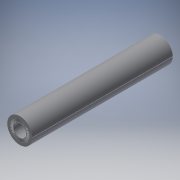
# Autodesk Inventor part: shtamp
Saved by Autodesk Inventor 2016 SP1 (Build 200210100, 210)
## iProperties
Created: 2017-07-05
Part Number: shtamp
Material: Типовые
Document SubType Name: Modeling
Designer: user
Density: 1 g/cm^3
Appearance: По умолчанию
Author: user
Autodesk Inventor part; units mm, degrees
ref_plane "YZ Plane" through (0, 0, 0) normal (1, 0, 0) x (0, 1, 0)
ref_plane "XZ Plane" through (0, 0, 0) normal (0, 1, 0) x (-1, 0, 0)
ref_plane "XY Plane" through (0, 0, 0) normal (0, 0, 1) x (1, 0, 0)
sketch "Эскиз1" plane through (0, 0, 0) normal (0, 1, 0) x (-1, 0, 0)
  arc A0 (-177.7324, -2.5) -> (-177.7324, 2.5) centre (0, 0) ccw
  circle A1 centre (0, 0) radius 90.075
  line L0 (134.775, -4.8) -> (97.375, -4.8)
  line L1 (92.575, 0) -> (92.575, 0)
  line L2 (97.375, 4.8) -> (134.775, 4.8)
  line L3 (139.575, 0) -> (139.575, 0)
  arc A2 (139.575, 0) -> (134.775, 4.8) centre (134.775, 0) ccw
  arc A3 (134.775, -4.8) -> (139.575, 0) centre (134.775, 0) ccw
  arc A4 (97.375, 4.8) -> (92.575, 0) centre (97.375, 0) ccw
  arc A5 (92.575, 0) -> (97.375, -4.8) centre (97.375, 0) ccw
  line L4 (95.9154, 17.4689) -> (132.9955, 22.3506)
  arc A6 (95.9154, 17.4689) -> (91.783, 12.0835) centre (96.5419, 12.71) ccw
  arc A7 (91.783, 12.0835) -> (97.1685, 7.9511) centre (96.5419, 12.71) ccw
  line L5 (134.2485, 12.8327) -> (97.1685, 7.9511)
  arc A8 (134.2485, 12.8327) -> (138.3809, 18.2182) centre (133.622, 17.5917) ccw
  arc A9 (138.3809, 18.2182) -> (132.9955, 22.3506) centre (133.622, 17.5917) ccw
  line L6 (92.8147, 29.8389) -> (128.9403, 39.5188)
  arc A10 (92.8147, 29.8389) -> (89.4206, 23.9602) centre (94.057, 25.2025) ccw
  arc A11 (89.4206, 23.9602) -> (95.2994, 20.5661) centre (94.057, 25.2025) ccw
  line L7 (131.425, 30.2459) -> (95.2994, 20.5661)
  arc A12 (131.425, 30.2459) -> (134.8191, 36.1247) centre (130.1827, 34.8823) ccw
  arc A13 (134.8191, 36.1247) -> (128.9403, 39.5188) centre (130.1827, 34.8823) ccw
  line L8 (88.1259, 41.6984) -> (122.679, 56.0108)
  arc A14 (88.1259, 41.6984) -> (85.5281, 35.4269) centre (89.9628, 37.2638) ccw
  arc A15 (85.5281, 35.4269) -> (91.7996, 32.8292) centre (89.9628, 37.2638) ccw
  line L9 (126.3527, 47.1415) -> (91.7996, 32.8292)
  arc A16 (126.3527, 47.1415) -> (128.9505, 53.413) centre (124.5159, 51.5762) ccw
  arc A17 (128.9505, 53.413) -> (122.679, 56.0108) centre (124.5159, 51.5762) ccw
  line L10 (81.9292, 52.8444) -> (114.3186, 71.5444)
  arc A18 (81.9292, 52.8444) -> (80.1723, 46.2875) centre (84.3292, 48.6875) ccw
  arc A19 (80.1723, 46.2875) -> (86.7292, 44.5306) centre (84.3292, 48.6875) ccw
  line L11 (119.1186, 63.2306) -> (86.7292, 44.5306)
  arc A20 (119.1186, 63.2306) -> (120.8755, 69.7875) centre (116.7186, 67.3875) ccw
  arc A21 (120.8755, 69.7875) -> (114.3186, 71.5444) centre (116.7186, 67.3875) ccw
  line L12 (74.3307, 63.0862) -> (104.0021, 85.8539)
  arc A22 (74.3307, 63.0862) -> (73.4447, 56.3561) centre (77.2528, 59.2781) ccw
  arc A23 (73.4447, 56.3561) -> (80.1748, 55.47) centre (77.2528, 59.2781) ccw
  line L13 (109.8463, 78.2377) -> (80.1748, 55.47)
  arc A24 (109.8463, 78.2377) -> (110.7323, 84.9679) centre (106.9242, 82.0458) ccw
  arc A25 (110.7323, 84.9679) -> (104.0021, 85.8539) centre (106.9242, 82.0458) ccw
  line L14 (65.4604, 72.2486) -> (91.9062, 98.6944)
  arc A26 (65.4604, 72.2486) -> (65.4604, 65.4604) centre (68.8545, 68.8545) ccw
  arc A27 (65.4604, 65.4604) -> (72.2486, 65.4604) centre (68.8545, 68.8545) ccw
  line L15 (98.6944, 91.9062) -> (72.2486, 65.4604)
  arc A28 (98.6944, 91.9062) -> (98.6944, 98.6944) centre (95.3003, 95.3003) ccw
  arc A29 (98.6944, 98.6944) -> (91.9062, 98.6944) centre (95.3003, 95.3003) ccw
  line L16 (55.47, 80.1748) -> (78.2377, 109.8463)
  arc A30 (55.47, 80.1748) -> (56.3561, 73.4447) centre (59.2781, 77.2528) ccw
  arc A31 (56.3561, 73.4447) -> (63.0862, 74.3307) centre (59.2781, 77.2528) ccw
  line L17 (85.8539, 104.0021) -> (63.0862, 74.3307)
  arc A32 (85.8539, 104.0021) -> (84.9679, 110.7323) centre (82.0458, 106.9242) ccw
  arc A33 (84.9679, 110.7323) -> (78.2377, 109.8463) centre (82.0458, 106.9242) ccw
  line L18 (44.5306, 86.7292) -> (63.2306, 119.1186)
  arc A34 (44.5306, 86.7292) -> (46.2875, 80.1723) centre (48.6875, 84.3292) ccw
  arc A35 (46.2875, 80.1723) -> (52.8444, 81.9292) centre (48.6875, 84.3292) ccw
  line L19 (71.5444, 114.3186) -> (52.8444, 81.9292)
  arc A36 (71.5444, 114.3186) -> (69.7875, 120.8755) centre (67.3875, 116.7186) ccw
  arc A37 (69.7875, 120.8755) -> (63.2306, 119.1186) centre (67.3875, 116.7186) ccw
  line L20 (32.8292, 91.7996) -> (47.1415, 126.3527)
  arc A38 (32.8292, 91.7996) -> (35.4269, 85.5281) centre (37.2638, 89.9628) ccw
  arc A39 (35.4269, 85.5281) -> (41.6984, 88.1259) centre (37.2638, 89.9628) ccw
  line L21 (56.0108, 122.679) -> (41.6984, 88.1259)
  arc A40 (56.0108, 122.679) -> (53.413, 128.9505) centre (51.5762, 124.5159) ccw
  arc A41 (53.413, 128.9505) -> (47.1415, 126.3527) centre (51.5762, 124.5159) ccw
  line L22 (20.5661, 95.2994) -> (30.2459, 131.425)
  arc A42 (20.5661, 95.2994) -> (23.9602, 89.4206) centre (25.2025, 94.057) ccw
  arc A43 (23.9602, 89.4206) -> (29.8389, 92.8147) centre (25.2025, 94.057) ccw
  line L23 (39.5188, 128.9403) -> (29.8389, 92.8147)
  arc A44 (39.5188, 128.9403) -> (36.1247, 134.8191) centre (34.8823, 130.1827) ccw
  arc A45 (36.1247, 134.8191) -> (30.2459, 131.425) centre (34.8823, 130.1827) ccw
  line L24 (7.9511, 97.1685) -> (12.8327, 134.2485)
  arc A46 (7.9511, 97.1685) -> (12.0835, 91.783) centre (12.71, 96.5419) ccw
  arc A47 (12.0835, 91.783) -> (17.4689, 95.9154) centre (12.71, 96.5419) ccw
  line L25 (22.3506, 132.9955) -> (17.4689, 95.9154)
  arc A48 (22.3506, 132.9955) -> (18.2182, 138.3809) centre (17.5917, 133.622) ccw
  arc A49 (18.2182, 138.3809) -> (12.8327, 134.2485) centre (17.5917, 133.622) ccw
  line L26 (-4.8, 97.375) -> (-4.8, 134.775)
  arc A50 (-4.8, 97.375) -> (0, 92.575) centre (0, 97.375) ccw
  arc A51 (0, 92.575) -> (4.8, 97.375) centre (0, 97.375) ccw
  line L27 (4.8, 134.775) -> (4.8, 97.375)
  arc A52 (4.8, 134.775) -> (0, 139.575) centre (0, 134.775) ccw
  arc A53 (0, 139.575) -> (-4.8, 134.775) centre (0, 134.775) ccw
  line L28 (-17.4689, 95.9154) -> (-22.3506, 132.9955)
  arc A54 (-17.4689, 95.9154) -> (-12.0835, 91.783) centre (-12.71, 96.5419) ccw
  arc A55 (-12.0835, 91.783) -> (-7.9511, 97.1685) centre (-12.71, 96.5419) ccw
  line L29 (-12.8327, 134.2485) -> (-7.9511, 97.1685)
  arc A56 (-12.8327, 134.2485) -> (-18.2182, 138.3809) centre (-17.5917, 133.622) ccw
  arc A57 (-18.2182, 138.3809) -> (-22.3506, 132.9955) centre (-17.5917, 133.622) ccw
  line L30 (-29.8389, 92.8147) -> (-39.5188, 128.9403)
  arc A58 (-29.8389, 92.8147) -> (-23.9602, 89.4206) centre (-25.2025, 94.057) ccw
  arc A59 (-23.9602, 89.4206) -> (-20.5661, 95.2994) centre (-25.2025, 94.057) ccw
  line L31 (-30.2459, 131.425) -> (-20.5661, 95.2994)
  arc A60 (-30.2459, 131.425) -> (-36.1247, 134.8191) centre (-34.8823, 130.1827) ccw
  arc A61 (-36.1247, 134.8191) -> (-39.5188, 128.9403) centre (-34.8823, 130.1827) ccw
  line L32 (-41.6984, 88.1259) -> (-56.0108, 122.679)
  arc A62 (-41.6984, 88.1259) -> (-35.4269, 85.5281) centre (-37.2638, 89.9628) ccw
  arc A63 (-35.4269, 85.5281) -> (-32.8292, 91.7996) centre (-37.2638, 89.9628) ccw
  line L33 (-47.1415, 126.3527) -> (-32.8292, 91.7996)
  arc A64 (-47.1415, 126.3527) -> (-53.413, 128.9505) centre (-51.5762, 124.5159) ccw
  arc A65 (-53.413, 128.9505) -> (-56.0108, 122.679) centre (-51.5762, 124.5159) ccw
  line L34 (-52.8444, 81.9292) -> (-71.5444, 114.3186)
  arc A66 (-52.8444, 81.9292) -> (-46.2875, 80.1723) centre (-48.6875, 84.3292) ccw
  arc A67 (-46.2875, 80.1723) -> (-44.5306, 86.7292) centre (-48.6875, 84.3292) ccw
  line L35 (-63.2306, 119.1186) -> (-44.5306, 86.7292)
  arc A68 (-63.2306, 119.1186) -> (-69.7875, 120.8755) centre (-67.3875, 116.7186) ccw
  arc A69 (-69.7875, 120.8755) -> (-71.5444, 114.3186) centre (-67.3875, 116.7186) ccw
  line L36 (-63.0862, 74.3307) -> (-85.8539, 104.0021)
  arc A70 (-63.0862, 74.3307) -> (-56.3561, 73.4447) centre (-59.2781, 77.2528) ccw
  arc A71 (-56.3561, 73.4447) -> (-55.47, 80.1748) centre (-59.2781, 77.2528) ccw
  line L37 (-78.2377, 109.8463) -> (-55.47, 80.1748)
  arc A72 (-78.2377, 109.8463) -> (-84.9679, 110.7323) centre (-82.0458, 106.9242) ccw
  arc A73 (-84.9679, 110.7323) -> (-85.8539, 104.0021) centre (-82.0458, 106.9242) ccw
  line L38 (-72.2486, 65.4604) -> (-98.6944, 91.9062)
  arc A74 (-72.2486, 65.4604) -> (-65.4604, 65.4604) centre (-68.8545, 68.8545) ccw
  arc A75 (-65.4604, 65.4604) -> (-65.4604, 72.2486) centre (-68.8545, 68.8545) ccw
  line L39 (-91.9062, 98.6944) -> (-65.4604, 72.2486)
  arc A76 (-91.9062, 98.6944) -> (-98.6944, 98.6944) centre (-95.3003, 95.3003) ccw
  arc A77 (-98.6944, 98.6944) -> (-98.6944, 91.9062) centre (-95.3003, 95.3003) ccw
  line L40 (-80.1748, 55.47) -> (-109.8463, 78.2377)
  arc A78 (-80.1748, 55.47) -> (-73.4447, 56.3561) centre (-77.2528, 59.2781) ccw
  arc A79 (-73.4447, 56.3561) -> (-74.3307, 63.0862) centre (-77.2528, 59.2781) ccw
  line L41 (-104.0021, 85.8539) -> (-74.3307, 63.0862)
  arc A80 (-104.0021, 85.8539) -> (-110.7323, 84.9679) centre (-106.9242, 82.0458) ccw
  arc A81 (-110.7323, 84.9679) -> (-109.8463, 78.2377) centre (-106.9242, 82.0458) ccw
  line L42 (-86.7292, 44.5306) -> (-119.1186, 63.2306)
  arc A82 (-86.7292, 44.5306) -> (-80.1723, 46.2875) centre (-84.3292, 48.6875) ccw
  arc A83 (-80.1723, 46.2875) -> (-81.9292, 52.8444) centre (-84.3292, 48.6875) ccw
  line L43 (-114.3186, 71.5444) -> (-81.9292, 52.8444)
  arc A84 (-114.3186, 71.5444) -> (-120.8755, 69.7875) centre (-116.7186, 67.3875) ccw
  arc A85 (-120.8755, 69.7875) -> (-119.1186, 63.2306) centre (-116.7186, 67.3875) ccw
  line L44 (-91.7996, 32.8292) -> (-126.3527, 47.1415)
  arc A86 (-91.7996, 32.8292) -> (-85.5281, 35.4269) centre (-89.9628, 37.2638) ccw
  arc A87 (-85.5281, 35.4269) -> (-88.1259, 41.6984) centre (-89.9628, 37.2638) ccw
  line L45 (-122.679, 56.0108) -> (-88.1259, 41.6984)
  arc A88 (-122.679, 56.0108) -> (-128.9505, 53.413) centre (-124.5159, 51.5762) ccw
  arc A89 (-128.9505, 53.413) -> (-126.3527, 47.1415) centre (-124.5159, 51.5762) ccw
  line L46 (-95.2994, 20.5661) -> (-131.425, 30.2459)
  arc A90 (-95.2994, 20.5661) -> (-89.4206, 23.9602) centre (-94.057, 25.2025) ccw
  arc A91 (-89.4206, 23.9602) -> (-92.8147, 29.8389) centre (-94.057, 25.2025) ccw
  line L47 (-128.9403, 39.5188) -> (-92.8147, 29.8389)
  arc A92 (-128.9403, 39.5188) -> (-134.8191, 36.1247) centre (-130.1827, 34.8823) ccw
  arc A93 (-134.8191, 36.1247) -> (-131.425, 30.2459) centre (-130.1827, 34.8823) ccw
  line L48 (-97.1685, 7.9511) -> (-134.2485, 12.8327)
  arc A94 (-97.1685, 7.9511) -> (-91.783, 12.0835) centre (-96.5419, 12.71) ccw
  arc A95 (-91.783, 12.0835) -> (-95.9154, 17.4689) centre (-96.5419, 12.71) ccw
  line L49 (-132.9955, 22.3506) -> (-95.9154, 17.4689)
  arc A96 (-132.9955, 22.3506) -> (-138.3809, 18.2182) centre (-133.622, 17.5917) ccw
  arc A97 (-138.3809, 18.2182) -> (-134.2485, 12.8327) centre (-133.622, 17.5917) ccw
  line L50 (-97.375, -4.8) -> (-134.775, -4.8)
  arc A98 (-97.375, -4.8) -> (-92.575, 0) centre (-97.375, 0) ccw
  arc A99 (-92.575, 0) -> (-97.375, 4.8) centre (-97.375, 0) ccw
  line L51 (-134.775, 4.8) -> (-97.375, 4.8)
  arc A100 (-134.775, 4.8) -> (-139.575, 0) centre (-134.775, 0) ccw
  arc A101 (-139.575, 0) -> (-134.775, -4.8) centre (-134.775, 0) ccw
  line L52 (-95.9154, -17.4689) -> (-132.9955, -22.3506)
  arc A102 (-95.9154, -17.4689) -> (-91.783, -12.0835) centre (-96.5419, -12.71) ccw
  arc A103 (-91.783, -12.0835) -> (-97.1685, -7.9511) centre (-96.5419, -12.71) ccw
  line L53 (-134.2485, -12.8327) -> (-97.1685, -7.9511)
  arc A104 (-134.2485, -12.8327) -> (-138.3809, -18.2182) centre (-133.622, -17.5917) ccw
  arc A105 (-138.3809, -18.2182) -> (-132.9955, -22.3506) centre (-133.622, -17.5917) ccw
  line L54 (-92.8147, -29.8389) -> (-128.9403, -39.5188)
  arc A106 (-92.8147, -29.8389) -> (-89.4206, -23.9602) centre (-94.057, -25.2025) ccw
  arc A107 (-89.4206, -23.9602) -> (-95.2994, -20.5661) centre (-94.057, -25.2025) ccw
  line L55 (-131.425, -30.2459) -> (-95.2994, -20.5661)
  arc A108 (-131.425, -30.2459) -> (-134.8191, -36.1247) centre (-130.1827, -34.8823) ccw
  arc A109 (-134.8191, -36.1247) -> (-128.9403, -39.5188) centre (-130.1827, -34.8823) ccw
  line L56 (-88.1259, -41.6984) -> (-122.679, -56.0108)
  arc A110 (-88.1259, -41.6984) -> (-85.5281, -35.4269) centre (-89.9628, -37.2638) ccw
  arc A111 (-85.5281, -35.4269) -> (-91.7996, -32.8292) centre (-89.9628, -37.2638) ccw
  line L57 (-126.3527, -47.1415) -> (-91.7996, -32.8292)
  arc A112 (-126.3527, -47.1415) -> (-128.9505, -53.413) centre (-124.5159, -51.5762) ccw
  arc A113 (-128.9505, -53.413) -> (-122.679, -56.0108) centre (-124.5159, -51.5762) ccw
  line L58 (-81.9292, -52.8444) -> (-114.3186, -71.5444)
  arc A114 (-81.9292, -52.8444) -> (-80.1723, -46.2875) centre (-84.3292, -48.6875) ccw
  arc A115 (-80.1723, -46.2875) -> (-86.7292, -44.5306) centre (-84.3292, -48.6875) ccw
  line L59 (-119.1186, -63.2306) -> (-86.7292, -44.5306)
  arc A116 (-119.1186, -63.2306) -> (-120.8755, -69.7875) centre (-116.7186, -67.3875) ccw
  arc A117 (-120.8755, -69.7875) -> (-114.3186, -71.5444) centre (-116.7186, -67.3875) ccw
  line L60 (-74.3307, -63.0862) -> (-104.0021, -85.8539)
  arc A118 (-74.3307, -63.0862) -> (-73.4447, -56.3561) centre (-77.2528, -59.2781) ccw
  arc A119 (-73.4447, -56.3561) -> (-80.1748, -55.47) centre (-77.2528, -59.2781) ccw
  line L61 (-109.8463, -78.2377) -> (-80.1748, -55.47)
  arc A120 (-109.8463, -78.2377) -> (-110.7323, -84.9679) centre (-106.9242, -82.0458) ccw
  arc A121 (-110.7323, -84.9679) -> (-104.0021, -85.8539) centre (-106.9242, -82.0458) ccw
  line L62 (-65.4604, -72.2486) -> (-91.9062, -98.6944)
  arc A122 (-65.4604, -72.2486) -> (-65.4604, -65.4604) centre (-68.8545, -68.8545) ccw
  arc A123 (-65.4604, -65.4604) -> (-72.2486, -65.4604) centre (-68.8545, -68.8545) ccw
  line L63 (-98.6944, -91.9062) -> (-72.2486, -65.4604)
  arc A124 (-98.6944, -91.9062) -> (-98.6944, -98.6944) centre (-95.3003, -95.3003) ccw
  arc A125 (-98.6944, -98.6944) -> (-91.9062, -98.6944) centre (-95.3003, -95.3003) ccw
  line L64 (-55.47, -80.1748) -> (-78.2377, -109.8463)
  arc A126 (-55.47, -80.1748) -> (-56.3561, -73.4447) centre (-59.2781, -77.2528) ccw
  arc A127 (-56.3561, -73.4447) -> (-63.0862, -74.3307) centre (-59.2781, -77.2528) ccw
  line L65 (-85.8539, -104.0021) -> (-63.0862, -74.3307)
  arc A128 (-85.8539, -104.0021) -> (-84.9679, -110.7323) centre (-82.0458, -106.9242) ccw
  arc A129 (-84.9679, -110.7323) -> (-78.2377, -109.8463) centre (-82.0458, -106.9242) ccw
  line L66 (-44.5306, -86.7292) -> (-63.2306, -119.1186)
  arc A130 (-44.5306, -86.7292) -> (-46.2875, -80.1723) centre (-48.6875, -84.3292) ccw
  arc A131 (-46.2875, -80.1723) -> (-52.8444, -81.9292) centre (-48.6875, -84.3292) ccw
  line L67 (-71.5444, -114.3186) -> (-52.8444, -81.9292)
  arc A132 (-71.5444, -114.3186) -> (-69.7875, -120.8755) centre (-67.3875, -116.7186) ccw
  arc A133 (-69.7875, -120.8755) -> (-63.2306, -119.1186) centre (-67.3875, -116.7186) ccw
  line L68 (-32.8292, -91.7996) -> (-47.1415, -126.3527)
  arc A134 (-32.8292, -91.7996) -> (-35.4269, -85.5281) centre (-37.2638, -89.9628) ccw
  arc A135 (-35.4269, -85.5281) -> (-41.6984, -88.1259) centre (-37.2638, -89.9628) ccw
  line L69 (-56.0108, -122.679) -> (-41.6984, -88.1259)
  arc A136 (-56.0108, -122.679) -> (-53.413, -128.9505) centre (-51.5762, -124.5159) ccw
  arc A137 (-53.413, -128.9505) -> (-47.1415, -126.3527) centre (-51.5762, -124.5159) ccw
  line L70 (-20.5661, -95.2994) -> (-30.2459, -131.425)
  arc A138 (-20.5661, -95.2994) -> (-23.9602, -89.4206) centre (-25.2025, -94.057) ccw
  arc A139 (-23.9602, -89.4206) -> (-29.8389, -92.8147) centre (-25.2025, -94.057) ccw
  line L71 (-39.5188, -128.9403) -> (-29.8389, -92.8147)
  arc A140 (-39.5188, -128.9403) -> (-36.1247, -134.8191) centre (-34.8823, -130.1827) ccw
  arc A141 (-36.1247, -134.8191) -> (-30.2459, -131.425) centre (-34.8823, -130.1827) ccw
  line L72 (-7.9511, -97.1685) -> (-12.8327, -134.2485)
  arc A142 (-7.9511, -97.1685) -> (-12.0835, -91.783) centre (-12.71, -96.5419) ccw
  arc A143 (-12.0835, -91.783) -> (-17.4689, -95.9154) centre (-12.71, -96.5419) ccw
  line L73 (-22.3506, -132.9955) -> (-17.4689, -95.9154)
  arc A144 (-22.3506, -132.9955) -> (-18.2182, -138.3809) centre (-17.5917, -133.622) ccw
  arc A145 (-18.2182, -138.3809) -> (-12.8327, -134.2485) centre (-17.5917, -133.622) ccw
  line L74 (4.8, -97.375) -> (4.8, -134.775)
  arc A146 (4.8, -97.375) -> (0, -92.575) centre (0, -97.375) ccw
  arc A147 (0, -92.575) -> (-4.8, -97.375) centre (0, -97.375) ccw
  line L75 (-4.8, -134.775) -> (-4.8, -97.375)
  arc A148 (-4.8, -134.775) -> (0, -139.575) centre (0, -134.775) ccw
  arc A149 (0, -139.575) -> (4.8, -134.775) centre (0, -134.775) ccw
  line L76 (17.4689, -95.9154) -> (22.3506, -132.9955)
  arc A150 (17.4689, -95.9154) -> (12.0835, -91.783) centre (12.71, -96.5419) ccw
  arc A151 (12.0835, -91.783) -> (7.9511, -97.1685) centre (12.71, -96.5419) ccw
  line L77 (12.8327, -134.2485) -> (7.9511, -97.1685)
  arc A152 (12.8327, -134.2485) -> (18.2182, -138.3809) centre (17.5917, -133.622) ccw
  arc A153 (18.2182, -138.3809) -> (22.3506, -132.9955) centre (17.5917, -133.622) ccw
  line L78 (29.8389, -92.8147) -> (39.5188, -128.9403)
  arc A154 (29.8389, -92.8147) -> (23.9602, -89.4206) centre (25.2025, -94.057) ccw
  arc A155 (23.9602, -89.4206) -> (20.5661, -95.2994) centre (25.2025, -94.057) ccw
  line L79 (30.2459, -131.425) -> (20.5661, -95.2994)
  arc A156 (30.2459, -131.425) -> (36.1247, -134.8191) centre (34.8823, -130.1827) ccw
  arc A157 (36.1247, -134.8191) -> (39.5188, -128.9403) centre (34.8823, -130.1827) ccw
  line L80 (41.6984, -88.1259) -> (56.0108, -122.679)
  arc A158 (41.6984, -88.1259) -> (35.4269, -85.5281) centre (37.2638, -89.9628) ccw
  arc A159 (35.4269, -85.5281) -> (32.8292, -91.7996) centre (37.2638, -89.9628) ccw
  line L81 (47.1415, -126.3527) -> (32.8292, -91.7996)
  arc A160 (47.1415, -126.3527) -> (53.413, -128.9505) centre (51.5762, -124.5159) ccw
  arc A161 (53.413, -128.9505) -> (56.0108, -122.679) centre (51.5762, -124.5159) ccw
  line L82 (52.8444, -81.9292) -> (71.5444, -114.3186)
  arc A162 (52.8444, -81.9292) -> (46.2875, -80.1723) centre (48.6875, -84.3292) ccw
  arc A163 (46.2875, -80.1723) -> (44.5306, -86.7292) centre (48.6875, -84.3292) ccw
  line L83 (63.2306, -119.1186) -> (44.5306, -86.7292)
  arc A164 (63.2306, -119.1186) -> (69.7875, -120.8755) centre (67.3875, -116.7186) ccw
  arc A165 (69.7875, -120.8755) -> (71.5444, -114.3186) centre (67.3875, -116.7186) ccw
  line L84 (63.0862, -74.3307) -> (85.8539, -104.0021)
  arc A166 (63.0862, -74.3307) -> (56.3561, -73.4447) centre (59.2781, -77.2528) ccw
  arc A167 (56.3561, -73.4447) -> (55.47, -80.1748) centre (59.2781, -77.2528) ccw
  line L85 (78.2377, -109.8463) -> (55.47, -80.1748)
  arc A168 (78.2377, -109.8463) -> (84.9679, -110.7323) centre (82.0458, -106.9242) ccw
  arc A169 (84.9679, -110.7323) -> (85.8539, -104.0021) centre (82.0458, -106.9242) ccw
  line L86 (72.2486, -65.4604) -> (98.6944, -91.9062)
  arc A170 (72.2486, -65.4604) -> (65.4604, -65.4604) centre (68.8545, -68.8545) ccw
  arc A171 (65.4604, -65.4604) -> (65.4604, -72.2486) centre (68.8545, -68.8545) ccw
  line L87 (91.9062, -98.6944) -> (65.4604, -72.2486)
  arc A172 (91.9062, -98.6944) -> (98.6944, -98.6944) centre (95.3003, -95.3003) ccw
  arc A173 (98.6944, -98.6944) -> (98.6944, -91.9062) centre (95.3003, -95.3003) ccw
  line L88 (80.1748, -55.47) -> (109.8463, -78.2377)
  arc A174 (80.1748, -55.47) -> (73.4447, -56.3561) centre (77.2528, -59.2781) ccw
  arc A175 (73.4447, -56.3561) -> (74.3307, -63.0862) centre (77.2528, -59.2781) ccw
  line L89 (104.0021, -85.8539) -> (74.3307, -63.0862)
  arc A176 (104.0021, -85.8539) -> (110.7323, -84.9679) centre (106.9242, -82.0458) ccw
  arc A177 (110.7323, -84.9679) -> (109.8463, -78.2377) centre (106.9242, -82.0458) ccw
  line L90 (86.7292, -44.5306) -> (119.1186, -63.2306)
  arc A178 (86.7292, -44.5306) -> (80.1723, -46.2875) centre (84.3292, -48.6875) ccw
  arc A179 (80.1723, -46.2875) -> (81.9292, -52.8444) centre (84.3292, -48.6875) ccw
  line L91 (114.3186, -71.5444) -> (81.9292, -52.8444)
  arc A180 (114.3186, -71.5444) -> (120.8755, -69.7875) centre (116.7186, -67.3875) ccw
  arc A181 (120.8755, -69.7875) -> (119.1186, -63.2306) centre (116.7186, -67.3875) ccw
  line L92 (91.7996, -32.8292) -> (126.3527, -47.1415)
  arc A182 (91.7996, -32.8292) -> (85.5281, -35.4269) centre (89.9628, -37.2638) ccw
  arc A183 (85.5281, -35.4269) -> (88.1259, -41.6984) centre (89.9628, -37.2638) ccw
  line L93 (122.679, -56.0108) -> (88.1259, -41.6984)
  arc A184 (122.679, -56.0108) -> (128.9505, -53.413) centre (124.5159, -51.5762) ccw
  arc A185 (128.9505, -53.413) -> (126.3527, -47.1415) centre (124.5159, -51.5762) ccw
  line L94 (95.2994, -20.5661) -> (131.425, -30.2459)
  arc A186 (95.2994, -20.5661) -> (89.4206, -23.9602) centre (94.057, -25.2025) ccw
  arc A187 (89.4206, -23.9602) -> (92.8147, -29.8389) centre (94.057, -25.2025) ccw
  line L95 (128.9403, -39.5188) -> (92.8147, -29.8389)
  arc A188 (128.9403, -39.5188) -> (134.8191, -36.1247) centre (130.1827, -34.8823) ccw
  arc A189 (134.8191, -36.1247) -> (131.425, -30.2459) centre (130.1827, -34.8823) ccw
  line L96 (97.1685, -7.9511) -> (134.2485, -12.8327)
  arc A190 (97.1685, -7.9511) -> (91.783, -12.0835) centre (96.5419, -12.71) ccw
  arc A191 (91.783, -12.0835) -> (95.9154, -17.4689) centre (96.5419, -12.71) ccw
  line L97 (132.9955, -22.3506) -> (95.9154, -17.4689)
  arc A192 (132.9955, -22.3506) -> (138.3809, -18.2182) centre (133.622, -17.5917) ccw
  arc A193 (138.3809, -18.2182) -> (134.2485, -12.8327) centre (133.622, -17.5917) ccw
  line L98 (-172.55, 2.5) -> (-177.7324, 2.5)
  line L99 (-177.7324, -2.5) -> (-172.55, -2.5)
  line L100 (-172.55, -2.5) -> (-172.55, 2.5)
  dimension "d0" = 355.5
  dimension "d1" = 180.15
  dimension "d2" = 92.575
  dimension "d4" = 4.8
  dimension "d5" = 4.8
  dimension "d6" = 47
  dimension "d7" = 4.8
  dimension "d8" = 4.8
  dimension "d9" = 4.8
  dimension "d10" = 4.8
  dimension "d13" = 360
  dimension "d15" = 2.5
  dimension "d16" = 2.5
  dimension "d17" = 5.2
  constraints: 386 point on circle, 202 end point, 194 centre point, 8 tangent, 3 parallel, 2 coincident, 2 horizontal, 1 perpendicular, 865 other
  measures "d0" diameter of A0
  measures "d1" diameter of A1
  measures "d2" distance from line of point (0, 0) L1
  measures "d4" distance from line of A1.centre L0
  measures "d5" distance from line of A1.centre L2
  measures "d6" distance between parallel lines of L3 L1
  measures "d7" radius of A2
  measures "d8" radius of A3
  measures "d9" radius of A4
  measures "d10" radius of A5
  measures "d15" distance from line of A0.centre L98
  measures "d16" distance from line of A0.centre L99
  measures "d17" distance edge to line of A0 L100
extrude "Выдавливание2" add sketch "Эскиз1" along normal blind 2000 contours L99 L100 L98 A0 | L0 A5 A4 L2 A2 A3 | L4 A9 A8 L5 A7 A6 | L6 A13 A12 L7 A11 A10 | L8 A17 A16 L9 A15 A14 | L10 A21 A20 L11 A19 A18 | L12 A25 A24 L13 A23 A22 | L14 A29 A28 L15 A27 A26 | L16 A33 A32 L17 A31 A30 | L18 A37 A36 L19 A35 A34 | L20 A41 A40 L21 A39 A38 | L22 A45 A44 L23 A43 A42 | L24 A49 A48 L25 A47 A46 | L26 A53 A52 L27 A51 A50 | L28 A57 A56 L29 A55 A54 | L30 A61 A60 L31 A59 A58 | L32 A65 A64 L33 A63 A62 | L34 A69 A68 L35 A67 A66 | L36 A73 A72 L37 A71 A70 | L38 A77 A76 L39 A75 A74 | L40 A81 A80 L41 A79 A78 | L42 A85 A84 L43 A83 A82 | L44 A89 A88 L45 A87 A86 | L46 A93 A92 L47 A91 A90 | L48 A97 A96 L49 A95 A94 | L50 A101 A100 L51 A99 A98 | L52 A105 A104 L53 A103 A102 | L54 A109 A108 L55 A107 A106 | L56 A113 A112 L57 A111 A110 | L58 A117 A116 L59 A115 A114 | L60 A121 A120 L61 A119 A118 | L62 A125 A124 L63 A123 A122 | L64 A129 A128 L65 A127 A126 | L66 A133 A132 L67 A131 A130 | L68 A137 A136 L69 A135 A134 | L70 A141 A140 L71 A139 A138 | L72 A145 A144 L73 A143 A142 | L74 A149 A148 L75 A147 A146 | L76 A153 A152 L77 A151 A150 | L78 A157 A156 L79 A155 A154 | L80 A161 A160 L81 A159 A158 | L82 A165 A164 L83 A163 A162 | L84 A169 A168 L85 A167 A166 | L86 A173 A172 L87 A171 A170 | L88 A177 A176 L89 A175 A174 | L90 A181 A180 L91 A179 A178 | L92 A185 A184 L93 A183 A182 | L94 A189 A188 L95 A187 A186 | L96 A193 A192 L97 A191 A190
extrude "Выдавливание3" cut sketch "Эскиз1" along normal blind 2000 contours L0 A5 A4 L2 A2 A3
pattern_circular "Круговой массив1" count 48 over 360 about axis through (0, 0, 0) along (0, 1, 0) of "Выдавливание3"
